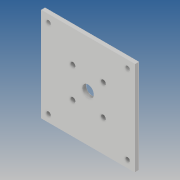
# Autodesk Inventor part: lazy susan5
Saved by Autodesk Inventor 2018 (Build 220112000, 112)
## iProperties
Created: 2017-11-17
Part Number: lazy susan5
Material: Generic
Document SubType Name: Modeling
Designer: 10283
Density: 1 g/cm^3
Appearance: Default
Author: 10283
Autodesk Inventor part; units mm, degrees
ref_plane "YZ Plane" through (0, 0, 0) normal (1, 0, 0) x (0, 1, 0)
ref_plane "XZ Plane" through (0, 0, 0) normal (0, 1, 0) x (-1, 0, 0)
ref_plane "XY Plane" through (0, 0, 0) normal (0, 0, 1) x (1, 0, 0)
sketch "Sketch1" plane through (0, 0, 0) normal (0, 0, 1) x (1, 0, 0)
  line L0 (-6.3269, 6.7325) -> (69.8731, 6.7325)
  line L1 (69.8731, 6.7325) -> (69.8731, -69.4675)
  line L2 (69.8731, -69.4675) -> (-6.3269, -69.4675)
  line L3 (-6.3269, -69.4675) -> (-6.3269, 6.7325)
  line L4 (-6.3269, 6.7325) -> (69.8731, -69.4675) construction
  line L5 (69.8731, 6.7325) -> (-6.3269, -69.4675) construction
  circle A0 centre (31.7731, -31.3675) radius 4.7625
  circle A1 centre (63.9041, 0.7635) radius 1.8161
  circle A2 centre (63.9041, -63.4985) radius 1.8161
  circle A3 centre (-0.3579, -63.4985) radius 1.8161
  circle A4 centre (-0.3579, 0.7635) radius 1.8161
  line L6 (12.7231, -50.4175) -> (50.8231, -50.4175) construction
  line L7 (50.8231, -50.4175) -> (50.8231, -12.3175) construction
  line L8 (50.8231, -12.3175) -> (12.7231, -12.3175) construction
  line L9 (12.7231, -12.3175) -> (12.7231, -50.4175) construction
  line L10 (12.7231, -50.4175) -> (50.8231, -12.3175) construction
  line L11 (50.8231, -50.4175) -> (12.7231, -12.3175) construction
  circle A5 centre (19.416, -19.0104) radius 2.0193
  circle A6 centre (44.1302, -19.0104) radius 2.0193
  circle A7 centre (19.416, -43.7246) radius 2.0193
  circle A8 centre (44.1302, -43.7246) radius 2.0193
  dimension "d0" = 76.2
  dimension "d1" = 76.2
  dimension "d2" = 9.525
  dimension "d4" = 3.6322
  dimension "d5" = 3.6322
  dimension "d6" = 3.6322
  dimension "d7" = 3.6322
  dimension "d11" = 38.1
  dimension "d12" = 38.1
  dimension "d13" = 4.0386
  dimension "d14" = 4.0386
  dimension "d15" = 4.0386
  dimension "d16" = 4.0386
  dimension "d17" = 24.7142
  dimension "d18" = 64.262
  constraints: 24 end point, 9 centre point, 8 point on line, 4 parallel, 4 vertical alignment, 3 horizontal alignment, 3 midpoint, 2 horizontal, 2 perpendicular, 1 coincident
  measures "d0" distance of L1.end L2.end
  measures "d1" distance of L0.end L1.end
  measures "d2" diameter of A0
  measures "d4" diameter of A1
  measures "d5" diameter of A2
  measures "d6" diameter of A3
  measures "d7" diameter of A4
  measures "d11" distance of L8.end L7.end
  measures "d12" distance of L6.end L7.end
  measures "d13" diameter of A5
  measures "d14" diameter of A6
  measures "d15" diameter of A7
  measures "d16" diameter of A8
  measures "d17" distance of A6.centre A5.centre
  measures "d18" distance of A1.centre A4.centre
extrude "Extrusion1" add sketch "Sketch1" along normal blind 3.175
body "Solid1"
